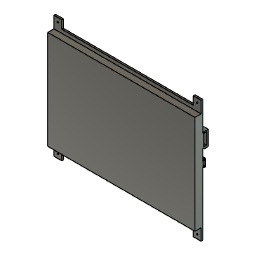
MockFrontPanel v5 (Autodesk Fusion 360 archive; units mm, degrees)
design "TouchScreen"
Autodesk Fusion 360 part; units mm, degrees
sketch "Sketch1" plane through (0, 0, 0) normal (0, 1, 0) x (1, 0, 0)
  line L0 (0, 0) -> (149, 0)
  line L1 (149, 0) -> (149, -107)
  line L2 (0, 0) -> (0, -107)
  line L3 (0, -107) -> (149, -107)
  line L4 (0, -107) -> (0, -115.3)
  line L5 (0, -115.3) -> (8, -115.3)
  line L6 (8, -115.3) -> (8, -107)
  line L7 (149, -107) -> (149, -115.3)
  line L8 (149, -115.3) -> (141, -115.3)
  line L9 (141, -115.3) -> (141, -107)
  line L10 (141, -107) -> (149, -115.3) construction
  line L11 (141, -115.3) -> (149, -107) construction
  circle A0 centre (145, -111.15) radius 0.75
  circle A1 centre (4, -111.15) radius 0.75
  line L12 (0, -115.3) -> (8, -107) construction
  line L13 (8, -115.3) -> (0, -107) construction
  line L14 (0, 0) -> (0, 8.3)
  line L15 (0, 8.3) -> (8, 8.3)
  line L16 (8, 8.3) -> (8, 0)
  line L17 (149, 0) -> (149, 8.3)
  line L18 (149, 8.3) -> (141, 8.3)
  line L19 (141, 8.3) -> (141, 0)
  line L20 (149, 0) -> (141, 8.3) construction
  line L21 (141, 0) -> (149, 8.3) construction
  line L22 (0, 0) -> (8, 8.3) construction
  line L23 (8, 0) -> (0, 8.3) construction
  circle A2 centre (4, 4.15) radius 0.75
  circle A3 centre (145, 4.15) radius 0.75
  dimension "d1" = 149
  dimension "d2" = 107
  dimension "d3" = 107
  dimension "d4" = 149
  dimension "d5" = 8.3
  dimension "d6" = 8
  dimension "d7" = 8.3
  dimension "d8" = 8
  dimension "d9" = 1.5
  dimension "d10" = 1.5
  dimension "d11" = 8.3
  dimension "d12" = 8
  dimension "d13" = 8.3
  dimension "d14" = 8
  dimension "d15" = 1.5
  dimension "d16" = 1.5
  constraint coincident L0.start L2.start
  constraint horizontal L0
  constraint perpendicular L0 L1
  constraint horizontal L3
  constraint perpendicular L3 L4
  constraint perpendicular L4 L5
  constraint coincident L3 L6.end
  constraint perpendicular L3 L6
  constraint perpendicular L3 L7
  constraint perpendicular L7 L8
  constraint coincident L3 L9.end
  constraint perpendicular L3 L9
  constraint midpoint L10 A0.centre
  constraint perpendicular L0 L14
  constraint perpendicular L14 L15
  constraint coincident L0 L16.end
  constraint perpendicular L0 L16
  constraint perpendicular L0 L17
  constraint perpendicular L17 L18
  constraint coincident L0 L19.end
  constraint perpendicular L0 L19
  constraint parallel L21 L22
  constraint midpoint L22 A2.centre
  constraint midpoint L21 A3.centre
  measures "d1" distance of L0.start L0.end
  measures "d2" distance of L0.end L1.end
  measures "d3" distance of L2.end L0.start
  measures "d4" distance of L2.end L1.end
  measures "d5" distance of L2.end L4.end
  measures "d6" distance of L4.end L5.end
  measures "d7" distance of L1.end L7.end
  measures "d8" distance of L7.end L8.end
  measures "d9" diameter of A0
  measures "d10" diameter of A1
  measures "d11" distance of L0.start L14.end
  measures "d12" distance of L14.end L15.end
  measures "d13" distance of L0.end L17.end
  measures "d14" distance of L17.end L18.end
  measures "d15" diameter of A2
  measures "d16" diameter of A3
extrude "Extrude1" add sketch "Sketch1" against normal blind 1.65
sketch "Sketch2" plane through (0, -1.65, 0) normal (0, -1, 0) x (1, 0, 0)
  circle A0 centre (145, -4.15) radius 0.75
  circle A1 centre (4, 111.15) radius 0.75
  circle A2 centre (145, 111.15) radius 0.75
  circle A3 centre (4, -4.15) radius 0.75
  line L0 (149, -8.3) -> (149, 115.3)
  line L1 (149, 115.3) -> (141, 115.3)
  line L2 (141, 115.3) -> (141, 107)
  line L3 (141, 107) -> (8, 107)
  line L4 (8, 107) -> (8, 115.3)
  line L5 (8, 115.3) -> (0, 115.3)
  line L6 (0, 115.3) -> (0, -8.3)
  line L7 (0, -8.3) -> (8, -8.3)
  line L8 (8, -8.3) -> (8, 0)
  line L9 (8, 0) -> (141, 0)
  line L10 (141, 0) -> (141, -8.3)
  line L11 (141, -8.3) -> (149, -8.3)
  line L12 (0, 107) -> (0, 103.4) construction
  line L13 (0, 103.4) -> (149, 103.4)
  line L14 (0, 0) -> (0, 3.6) construction
  line L15 (8, 107) -> (-0.0006, 107) construction
  line L16 (8, 0) -> (0, 0) construction
  line L17 (0, 3.6) -> (149, 3.6)
  dimension "d19" = 3.6
  dimension "d20" = 3.6
  constraint coincident L6 L12.start
  constraint coincident L0 L13.end
  constraint perpendicular L0 L13
  constraint coincident L14.start L16.end
  constraint perpendicular L9 L14
  constraint horizontal L15
  constraint coincident L3.end L4.start
  constraint coincident L8.end L9.start
  constraint coincident L0 L17.end
  constraint perpendicular L0 L17
  measures "d19" distance of L12.start L12.end
  measures "d20" distance of L14.start L14.end
extrude "Extrude2" add sketch "Sketch2" along normal blind 6.3 contours L0 L6 L13 L17
sketch "Sketch3" plane through (149, 0, 0) normal (1, 0, 0) x (0, 1, 0)
  line L0 (0, -8.3) -> (0, 115.3)
  line L1 (0, 115.3) -> (-1.65, 115.3)
  line L2 (-1.65, 115.3) -> (-1.65, 103.4)
  line L3 (-1.65, 103.4) -> (-7.95, 103.4)
  line L4 (-7.95, 103.4) -> (-7.95, 3.6)
  line L5 (-7.95, 3.6) -> (-1.65, 3.6)
  line L6 (-1.65, 3.6) -> (-1.65, -8.3)
  line L7 (-1.65, -8.3) -> (0, -8.3)
sketch "Sketch4" plane through (0, 0, 0) normal (0, 1, 0) x (-1, 0, 0)
  circle A0 centre (-145, -4.15) radius 0.75
  circle A1 centre (-4, 111.15) radius 0.75
  circle A2 centre (-145, 111.15) radius 0.75
  circle A3 centre (-4, -4.15) radius 0.75
  line L0 (-149, 115.3) -> (-149, -8.3)
  line L1 (-149, -8.3) -> (-141, -8.3)
  line L2 (-141, -8.3) -> (-141, 0)
  line L3 (-141, 0) -> (-8, 0)
  line L4 (-8, 0) -> (-8, -8.3)
  line L5 (-8, -8.3) -> (0, -8.3)
  line L6 (0, -8.3) -> (0, 115.3)
  line L7 (0, 115.3) -> (-8, 115.3)
  line L8 (-8, 115.3) -> (-8, 107)
  line L9 (-8, 107) -> (-141, 107)
  line L10 (-141, 107) -> (-141, 115.3)
  line L11 (-141, 115.3) -> (-149, 115.3)
  line L12 (-149, 106.8976) -> (-149, 86.2976) construction
  line L13 (-149, 86.2976) -> (-137, 86.2976)
  line L14 (-137, 86.2976) -> (-137, 71.0976)
  line L15 (-137, 71.0976) -> (-149, 71.0976)
  dimension "d23" = 20.6
  dimension "d24" = 12
  dimension "d25" = 15.2
  constraint coincident L0 L12.start
  constraint perpendicular L0 L13
  constraint perpendicular L13 L14
  constraint coincident L0 L15.end
  constraint perpendicular L0 L15
  measures "d23" distance of L12.start L12.end
  measures "d24" distance of L12.end L13.end
  measures "d25" distance of L13.end L14.end
extrude "Extrude3" add sketch "Sketch4" along normal blind 5.6 contours L0 L13 L14 L15
sketch "Sketch5" plane through (149, 0, 0) normal (1, 0, 0) x (0, 1, 0)
  line L0 (0, -8.3) -> (0, 71.0976)
  line L1 (0, 71.0976) -> (5.6, 71.0976)
  line L2 (5.6, 71.0976) -> (5.6, 86.2976)
  line L3 (5.6, 86.2976) -> (0, 86.2976)
  line L4 (0, 86.2976) -> (0, 115.3)
  line L5 (0, 115.3) -> (-1.65, 115.3)
  line L6 (-1.65, 115.3) -> (-1.65, 103.4)
  line L7 (-1.65, 103.4) -> (-7.95, 103.4)
  line L8 (-7.95, 103.4) -> (-7.95, 3.6)
  line L9 (-7.95, 3.6) -> (-1.65, 3.6)
  line L10 (-1.65, 3.6) -> (-1.65, -8.3)
  line L11 (-1.65, -8.3) -> (0, -8.3)
  line L12 (0, 86.2976) -> (0, 71.0976)
  line L13 (0, 86.2976) -> (0, 85.5476) construction
  arc A0 (0, 85.5476) -> (1.1901, 86.2976) centre (0.2339, 86.4956) ccw
  line L14 (0, 71.0976) -> (0, 71.8476) construction
  arc A1 (1.4983, 71.0976) -> (0, 71.8476) centre (0.1697, 70.3149) ccw
  dimension "d29" = 0.75
  dimension "d30" = 0.75
  constraint coincident L3.end L4.start
  constraint coincident L0.end L1.start
  constraint perpendicular L3 L13
  constraint coincident L3 A0.end
  constraint perpendicular L1 L14
  constraint coincident L1 A1.start
  measures "d29" distance of L3.end L13.end
  measures "d30" distance of L0.end L14.end
extrude "Extrude4" cut sketch "Sketch5" against normal blind 4 contours L1 L12 A1 | L3 L12 A0
sketch "Sketch6" plane through (149, 0, 0) normal (1, 0, 0) x (0, 1, 0)
  arc A0 (0, 85.5476) -> (1.1901, 86.2976) centre (0.2339, 86.4956) ccw
  line L0 (0, 85.5476) -> (0, 115.3)
  line L1 (0, 115.3) -> (-1.65, 115.3)
  line L2 (-1.65, 115.3) -> (-1.65, 103.4)
  line L3 (-1.65, 103.4) -> (-7.95, 103.4)
  line L4 (-7.95, 103.4) -> (-7.95, 3.6)
  line L5 (-7.95, 3.6) -> (-1.65, 3.6)
  line L6 (-1.65, 3.6) -> (-1.65, -8.3)
  line L7 (-1.65, -8.3) -> (0, -8.3)
  line L8 (0, -8.3) -> (0, 71.8476)
  arc A1 (1.4983, 71.0976) -> (0, 71.8476) centre (0.1697, 70.3149) ccw
  line L9 (1.4983, 71.0976) -> (5.6, 71.0976)
  line L10 (5.6, 71.0976) -> (5.6, 86.2976)
  line L11 (5.6, 86.2976) -> (1.1901, 86.2976)
  line L12 (1, 85) -> (1, 73)
  line L13 (1, 73) -> (4, 73)
  line L14 (4, 73) -> (4, 85)
  line L15 (4, 85) -> (1, 85)
  constraint vertical L12
  constraint perpendicular L12 L13
  constraint perpendicular L13 L14
  constraint perpendicular L12 L15
extrude "Extrude5" cut sketch "Sketch6" against normal blind 10 contours L12 L13 L14 L15
sketch "Sketch7" plane through (0, 0, 86.2976) normal (0, 0, 1) x (-1, 0, 0)
  line L0 (-145, 0) -> (-145, -1.1901)
  line L1 (-145, -1.1901) -> (-149, -1.1901)
  line L2 (-149, -1.1901) -> (-149, -5.6)
  line L3 (-149, -5.6) -> (-137, -5.6)
  line L4 (-137, -5.6) -> (-137, 0)
  line L5 (-137, 0) -> (-145, 0)
sketch "Sketch8" plane through (0, 0, 0) normal (0, 1, 0) x (-1, 0, 0)
  line L0 (-137, 71.0976) -> (-145, 71.0976)
  line L1 (-145, 71.0976) -> (-145, 71.8476)
  line L2 (-145, 71.8476) -> (-149, 71.8476)
  line L3 (-149, 71.8476) -> (-149, -8.3)
  line L4 (-149, -8.3) -> (-141, -8.3)
  line L5 (-141, -8.3) -> (-141, 0)
  line L6 (-141, 0) -> (-8, 0)
  line L7 (-8, 0) -> (-8, -8.3)
  line L8 (-8, -8.3) -> (0, -8.3)
  line L9 (0, -8.3) -> (0, 115.3)
  line L10 (0, 115.3) -> (-8, 115.3)
  line L11 (-8, 115.3) -> (-8, 107)
  line L12 (-8, 107) -> (-141, 107)
  line L13 (-141, 107) -> (-141, 115.3)
  line L14 (-141, 115.3) -> (-149, 115.3)
  line L15 (-149, 115.3) -> (-149, 85.5476)
  line L16 (-149, 85.5476) -> (-145, 85.5476)
  line L17 (-145, 85.5476) -> (-145, 86.2976)
  line L18 (-145, 86.2976) -> (-137, 86.2976)
  line L19 (-137, 86.2976) -> (-137, 71.0976)
  circle A0 centre (-145, -4.15) radius 0.75
  circle A1 centre (-4, 111.15) radius 0.75
  circle A2 centre (-145, 111.15) radius 0.75
  circle A3 centre (-4, -4.15) radius 0.75
  line L20 (-149, 71.0976) -> (-149, 62.1976) construction
  line L21 (-149, 62.1976) -> (-143.7, 62.1976)
  line L22 (-143.7, 62.1976) -> (-143.7, 54.5976)
  line L23 (-143.7, 54.5976) -> (-149, 54.5976)
  dimension "d35" = 8.9
  dimension "d36" = 5.3
  dimension "d37" = 7.6
  constraint coincident L3 L20.start
  constraint perpendicular L0 L20
  constraint perpendicular L20 L21
  constraint perpendicular L21 L22
  constraint coincident L3 L23.end
  constraint perpendicular L3 L23
  measures "d35" distance of L20.start L20.end
  measures "d36" distance of L20.end L21.end
  measures "d37" distance of L21.end L22.end
extrude "Extrude6" add sketch "Sketch8" along normal blind 2.75 contours L3 L21 L22 L23
sketch "Sketch9" plane through (149, 0, 0) normal (1, 0, 0) x (0, 1, 0)
  line L0 (1, 73) -> (1, 85)
  line L1 (1, 85) -> (4, 85)
  line L2 (4, 85) -> (4, 73)
  line L3 (4, 73) -> (1, 73)
  arc A0 (0, 85.5476) -> (1.1901, 86.2976) centre (0.2339, 86.4956) ccw
  line L4 (0, 85.5476) -> (0, 115.3)
  line L5 (0, 115.3) -> (-1.65, 115.3)
  line L6 (-1.65, 115.3) -> (-1.65, 103.4)
  line L7 (-1.65, 103.4) -> (-7.95, 103.4)
  line L8 (-7.95, 103.4) -> (-7.95, 3.6)
  line L9 (-7.95, 3.6) -> (-1.65, 3.6)
  line L10 (-1.65, 3.6) -> (-1.65, -8.3)
  line L11 (-1.65, -8.3) -> (0, -8.3)
  line L12 (0, -8.3) -> (0, 54.5976)
  line L13 (0, 54.5976) -> (2.75, 54.5976)
  line L14 (2.75, 54.5976) -> (2.75, 62.1976)
  line L15 (2.75, 62.1976) -> (0, 62.1976)
  line L16 (0, 62.1976) -> (0, 71.8476)
  arc A1 (1.4983, 71.0976) -> (0, 71.8476) centre (0.1697, 70.3149) ccw
  line L17 (1.4983, 71.0976) -> (5.6, 71.0976)
  line L18 (5.6, 71.0976) -> (5.6, 86.2976)
  line L19 (5.6, 86.2976) -> (1.1901, 86.2976)
  line L20 (2.75, 62.1976) -> (0, 61.5)
  line L21 (2.75, 62.1976) -> (0, 61.5)
  line L22 (2.75, 54.5976) -> (0, 55.2952)
  line L23 (0, 62.1976) -> (0, 61.5)
  line L24 (0, 55.2952) -> (0, 54.5976)
  constraint coincident L14.end L15.start
  constraint coincident L15.end L16.start
  constraint perpendicular L15 L23
  constraint coincident L12.end L13.start
  constraint perpendicular L13 L24
extrude "Extrude7" cut sketch "Sketch9" against normal blind 1.1 contours L15 L20 L21 L23 | L13 L22 L24
sketch "Sketch10" plane through (149, 0, 0) normal (1, 0, 0) x (0, 1, 0)
  line L0 (1, 73) -> (1, 85)
  line L1 (1, 85) -> (4, 85)
  line L2 (4, 85) -> (4, 73)
  line L3 (4, 73) -> (1, 73)
  line L4 (0, -8.3) -> (0, 55.2952)
  line L5 (0, 55.2952) -> (2.75, 54.5976)
  line L6 (2.75, 54.5976) -> (2.75, 62.1976)
  line L7 (2.75, 62.1976) -> (0, 61.5)
  line L8 (0, 61.5) -> (0, 71.8476)
  arc A0 (1.4983, 71.0976) -> (0, 71.8476) centre (0.1697, 70.3149) ccw
  line L9 (1.4983, 71.0976) -> (5.6, 71.0976)
  line L10 (5.6, 71.0976) -> (5.6, 86.2976)
  line L11 (5.6, 86.2976) -> (1.1901, 86.2976)
  arc A1 (0, 85.5476) -> (1.1901, 86.2976) centre (0.2339, 86.4956) ccw
  line L12 (0, 85.5476) -> (0, 115.3)
  line L13 (0, 115.3) -> (-1.65, 115.3)
  line L14 (-1.65, 115.3) -> (-1.65, 103.4)
  line L15 (-1.65, 103.4) -> (-7.95, 103.4)
  line L16 (-7.95, 103.4) -> (-7.95, 3.6)
  line L17 (-7.95, 3.6) -> (-1.65, 3.6)
  line L18 (-1.65, 3.6) -> (-1.65, -8.3)
  line L19 (-1.65, -8.3) -> (0, -8.3)
  line L20 (0.3, 61) -> (2.4, 61)
  line L21 (2.4, 61) -> (2.4, 55.5)
  line L22 (2.4, 55.5) -> (0.5, 55.5)
  line L23 (0.5, 55.5) -> (0.3, 55.5)
  line L24 (0.3, 55.5) -> (0.3, 61)
  constraint perpendicular L6 L20
  constraint perpendicular L20 L21
  constraint perpendicular L21 L22
  constraint perpendicular L21 L23
  constraint perpendicular L20 L24
extrude "Extrude8" cut sketch "Sketch10" against normal blind 4.1 contours L20 L21 L22 L23 L24
